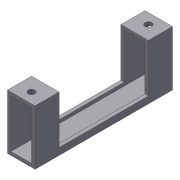
# Autodesk Inventor part: Frame_BatteryMount
Saved by Autodesk Inventor 2012 (Build 160160000, 160)
## iProperties
Created: 2012-01-17
Part Number: Frame_BatteryMount
Material: Aluminum-6061
Document SubType Name: Modeling
Designer: JesseK
Density: 2.71 g/cm^3
Mass: 75.4359 g
Surface Area: 197.58 cm^2
Volume: 27.8361 cm^3
Author: JesseK
Autodesk Inventor part; units mm, degrees
ref_plane "YZ Plane" through (0, 0, 0) normal (1, 0, 0) x (0, 1, 0)
ref_plane "XZ Plane" through (0, 0, 0) normal (0, 1, 0) x (-1, 0, 0)
ref_plane "XY Plane" through (0, 0, 0) normal (0, 0, 1) x (1, 0, 0)
sketch "Sketch1" plane through (0, 0, 0) normal (0, 0, 1) x (1, 0, 0)
  line L0 (0, 0) -> (25.4, 0)
  line L1 (25.4, 0) -> (25.4, 50.8)
  line L2 (25.4, 50.8) -> (0, 50.8)
  line L3 (0, 50.8) -> (0, 0)
  dimension "d0" = 25.4
  dimension "d1" = 50.8
  constraints: 8 end point, 2 parallel, 1 horizontal, 1 perpendicular
  measures "d0" distance of L1.end L2.end
  measures "d1" distance of L0.end L1.end
extrude "Extrusion1" add sketch "Sketch1" along normal blind 127
shell "Shell1" thickness 3.175 removed faces 2 at (8.4667, 33.8667, 0) at (8.4667, 33.8667, 127)
sketch "Sketch3" plane through (0, 50.8, 0) normal (0, 1, 0) x (1, 0, 0)
  line L0 (0, -127) -> (25.4, -127) projected
  line L1 (25.4, 0) -> (25.4, -127) projected
  line L2 (25.4, 0) -> (0, 0) projected
  line L3 (0, 0) -> (0, -127) projected
  circle A0 centre (12.7, -9.525) radius 3.175
  circle A1 centre (12.7, -117.475) radius 3.175
  dimension "d10" = 6.35
  dimension "d11" = 12.7
  dimension "d12" = 9.525
  dimension "d13" = 12.7
  dimension "d14" = 9.525
  constraints: 2 centre point, 1 equal radius
  measures "d10" diameter of A0
  measures "d11" distance from line of L3 A0.centre
  measures "d12" distance from line of L2 A0.centre
  measures "d13" distance from line of L1 A1.centre
  measures "d14" distance from line of L0 A1.centre
sketch "Sketch2" plane through (25.4, 0, 0) normal (1, 0, 0) x (0, 0, -1)
  line L0 (-127, 50.8) -> (-127, 0) projected
  line L1 (0, 0) -> (-127, 0) projected
  line L2 (0, 0) -> (0, 50.8) projected
  line L3 (0, 50.8) -> (-127, 50.8) projected
  line L4 (-104.775, 50.8) -> (-22.225, 50.8)
  line L5 (-22.225, 50.8) -> (-22.225, 6.35)
  line L6 (-22.225, 6.35) -> (-104.775, 6.35)
  line L7 (-104.775, 6.35) -> (-104.775, 50.8)
  line L8 (-22.225, 35.4291) -> (0, 35.4291) construction
  line L9 (-104.775, 35.4291) -> (-127, 35.4291) construction
  dimension "d5" = 6.35
  dimension "d19" = 82.55
  constraints: 12 end point, 5 point on line, 3 horizontal, 2 collinear, 2 parallel, 1 perpendicular
  measures "d5" distance between parallel lines of L1 L6
  measures "d19" distance of L5.end L6.end
extrude "Extrusion3" cut sketch "Sketch3" against normal up to next contours A0 | A1
extrude "Extrusion4" cut sketch "Sketch2" against normal through all contours L3 L5 L6 L7
body "Solid1"
